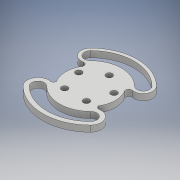
# Autodesk Inventor part: пр3дет1
Saved by Autodesk Inventor 2018 (Build 220112000, 112)
## iProperties
Created: 2020-04-07
Part Number: пр3дет1
Material: Типовые
Document SubType Name: Modeling
Designer: asus
Density: 1 g/cm^3
Appearance: По умолчанию
Author: asus
Autodesk Inventor part; units mm, degrees
ref_plane "YZ Plane" through (0, 0, 0) normal (1, 0, 0) x (0, 1, 0)
ref_plane "XZ Plane" through (0, 0, 0) normal (0, 1, 0) x (-1, 0, 0)
ref_plane "XY Plane" through (0, 0, 0) normal (0, 0, 1) x (1, 0, 0)
sketch "Эскиз1" plane through (0, 0, 0) normal (0, 0, 1) x (1, 0, 0)
  circle A0 centre (0, 0) radius 40
  circle A1 centre (0, 0) radius 30 construction
  line L0 (17.5791, -24.31) -> (-17.6879, -24.2309) construction
  line L1 (-17.6879, -24.2309) -> (-28.5108, 9.3345) construction
  line L2 (-28.5108, 9.3345) -> (0.0673, 29.9999) construction
  line L3 (0.0673, 29.9999) -> (28.5524, 9.2065) construction
  line L4 (28.5524, 9.2065) -> (17.5791, -24.31) construction
  circle A2 centre (-28.5108, 9.3345) radius 5
  circle A3 centre (0.0673, 29.9999) radius 5
  circle A4 centre (28.5524, 9.2065) radius 5
  circle A5 centre (17.5791, -24.31) radius 5
  circle A6 centre (-17.6879, -24.2309) radius 5
  circle A7 centre (0, 0) radius 60 construction
  line L5 (0, 0) -> (42.4264, 42.4264)
  line L6 (0, 0) -> (60, 0) construction
  line L7 (42.4264, 42.4264) -> (-42.4264, 42.4264) construction
  line L8 (-42.4264, 42.4264) -> (-42.4264, -42.4264) construction
  line L9 (42.4264, -42.4264) -> (42.4264, 42.4264) construction
  line L10 (-42.4264, -42.4264) -> (42.4264, -42.4264) construction
  arc A8 (42.4264, 42.4264) -> (-42.4264, 42.4264) centre (0, 0) ccw construction
  arc A9 (49.4975, 49.4975) -> (-49.4975, 49.4975) centre (0, 0) ccw
  arc A10 (35.3553, 35.3553) -> (-35.3553, 35.3553) centre (0, 0) ccw
  arc A11 (35.3553, 35.3553) -> (49.4975, 49.4975) centre (42.4264, 42.4264) ccw
  arc A12 (-49.4975, 49.4975) -> (-35.3553, 35.3553) centre (-42.4264, 42.4264) ccw
  arc A13 (42.4264, 42.4264) -> (-42.4264, 42.4264) centre (0, 0) ccw construction
  arc A14 (53.033, 53.033) -> (-53.033, 53.033) centre (0, 0) ccw
  arc A15 (-42.4264, -42.4264) -> (42.4264, -42.4264) centre (0, 0) ccw construction
  arc A16 (-49.4975, -49.4975) -> (49.4975, -49.4975) centre (0, 0) ccw
  arc A17 (-35.3553, -35.3553) -> (35.3553, -35.3553) centre (0, 0) ccw
  arc A18 (-35.3553, -35.3553) -> (-49.4975, -49.4975) centre (-42.4264, -42.4264) ccw
  arc A19 (49.4975, -49.4975) -> (35.3553, -35.3553) centre (42.4264, -42.4264) ccw
  arc A20 (-42.4264, -42.4264) -> (42.4264, -42.4264) centre (0, 0) ccw construction
  arc A21 (-54.4472, -54.4472) -> (54.4472, -54.4472) centre (0, 0) ccw
  arc A22 (-33.9116, 21.2132) -> (-39.6003, 27.695) centre (-38.6583, 22.7846) ccw
  arc A23 (39.6003, 27.695) -> (33.9116, 21.2132) centre (38.6583, 22.7846) ccw
  arc A24 (-38.6583, -25.8493) -> (-33.9116, -21.2132) centre (-38.8988, -20.8551) ccw
  arc A25 (33.9116, -21.2132) -> (38.6583, -25.8493) centre (38.8988, -20.8551) ccw
  arc A26 (-53.033, 53.033) -> (-39.6003, 27.695) centre (-42.4264, 42.4264) ccw
  arc A27 (39.6003, 27.695) -> (53.033, 53.033) centre (42.4264, 42.4264) ccw
  arc A28 (-38.6583, -25.8493) -> (-54.4472, -54.4472) centre (-42.4264, -42.4264) ccw
  arc A29 (54.4472, -54.4472) -> (38.6583, -25.8493) centre (42.4264, -42.4264) ccw
  dimension "d1" = 60
  dimension "d0" = 80
  dimension "d8" = 10
  dimension "d9" = 33.5165
  dimension "d22" = 120
  dimension "d23" = 60
  dimension "d24" = 45
  dimension "d25" = 20
  dimension "d27" = 20
  dimension "d29" = 5
  dimension "d31" = 5
  dimension "d32" = 5
  dimension "d33" = 5
  dimension "d34" = 2.8261
  dimension "d35" = 3.5276
  dimension "d36" = 20.8551
  dimension "d37" = 76.338
  dimension "d38" = 76.3381
  dimension "d39" = 81.0847
  dimension "d40" = 15
  dimension "d41" = 17
  constraints: 51 point on circle, 29 centre point, 22 end point, 16 tangent, 9 coincident, 6 equal radius, 4 concentric, 2 horizontal, 1 equal length, 1 parallel, 1 perpendicular, 14 other
  measures "d0" diameter of A0
  measures "d8" diameter of A4
  measures "d9" vertical distance of L3.end L0.start
  measures "d22" diameter of A7
  measures "d23" distance of L5.start L5.end
  measures "d24" angle of L6 L5
  measures "d25" diameter of A11
  measures "d27" diameter of A19
  measures "d29" radius of A22
  measures "d31" radius of A23
  measures "d32" radius of A24
  measures "d33" radius of A25
  measures "d34" distance from line of A23.start L9
  measures "d35" distance from line of A25.centre L9
  measures "d36" distance from line of A25.centre L6
  measures "d37" distance from line of A0.start L9
  measures "d38" distance from line of A24.end L9
  measures "d39" distance from line of A24.start L9
  measures "d40" radius of A27
  measures "d41" radius of A29
sketch "Эскиз2" plane through (0, 0, 0) normal (0, 0, 1) x (1, 0, 0)
  point P0 (0, 0)
extrude "Выдавливание1" add sketch "Эскиз1" along normal blind 10
